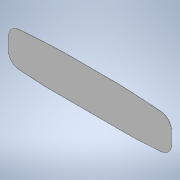
# Autodesk Inventor part: 7 Segment Clock Shell
Saved by Autodesk Inventor 2021 (Build 250183000, 183)
## iProperties
Created: 2020-06-27
Part Number: 7 Segment Clock Shell
Material: Generic
Document SubType Name: Modeling
Designer: dech3
Density: 1 g/cm^3
Appearance: Default
Author: dech3
Autodesk Inventor part; units mm, degrees
ref_plane "YZ Plane" through (0, 0, 0) normal (1, 0, 0) x (0, 1, 0)
ref_plane "XZ Plane" through (0, 0, 0) normal (0, 1, 0) x (-1, 0, 0)
ref_plane "XY Plane" through (0, 0, 0) normal (0, 0, 1) x (1, 0, 0)
sketch "Block1" plane through (0, 0, 0) normal (0, 0, 1) x (1, 0, 0)
  arc A0 (261.5609, 58.5131) -> (100.3256, 67.9894) centre (0, -3015.4231) ccw
  arc A1 (-100.3256, 67.9894) -> (-261.5609, 58.5131) centre (0, -3015.4231) ccw
  line L0 (-159.5034, -75) -> (159.5034, -75)
  arc A2 (-263.2612, -68.2167) -> (-160.4975, -74.9753) centre (0, 3150) ccw
  arc A3 (160.4975, -74.9753) -> (263.2612, -68.2167) centre (0, 3150) ccw
  arc A4 (300, 16.6643) -> (261.5609, 58.5131) centre (258, 16.6643) ccw
  arc A5 (263.2612, -68.2167) -> (300, -28.3498) centre (260, -28.3498) ccw
  arc A6 (-300, -28.3498) -> (-263.2612, -68.2167) centre (-260, -28.3498) ccw
  arc A7 (-261.5609, 58.5131) -> (-300, 16.6643) centre (-258, 16.6643) ccw
  arc A8 (-99.6752, 68) -> (-100.3256, 67.9894) centre (-99.6752, 48) ccw
  arc A9 (100.3256, 67.9894) -> (99.6752, 68) centre (99.6752, 48) ccw
  arc A10 (159.5034, -75) -> (160.4975, -74.9753) centre (159.5034, -55) ccw
  arc A11 (-160.4975, -74.9753) -> (-159.5034, -75) centre (-159.5034, -55) ccw
  line L1 (-99.6752, 68) -> (99.6752, 68)
  line L2 (300, 16.6643) -> (300, -28.3498)
  line L3 (-300, -28.3498) -> (-300, 16.6643)
  point P0 (0, -2.2582)
  point P1 (-300, 55)
  point P2 (300, 55)
  point P3 (-300, -65)
  point P4 (300, -65)
  point P5 (-160, -75)
  point P6 (160, -75)
  point P7 (-100, 68)
  point P8 (100, 68)
  dimension "d0" = 600
  dimension "d14" = 120
  dimension "d13" = 120
  dimension "d12" = 140
  dimension "d10" = 140
  dimension "d3" = 200
  dimension "d1" = 200
  dimension "d20" = 200
  dimension "d21" = 320
  dimension "d2" = 143
  dimension "d11" = 10
  dimension "d9" = 10
  dimension "d22" = 13
  dimension "d23" = 13
  dimension "d8" = 42
  dimension "d7" = 40
  dimension "d6" = 40
  dimension "d5" = 42
  dimension "d4" = 20
  measures "d0" distance between parallel lines of L2 L3
  measures "d14" distance of point (-300, 55) point (-300, -65)
  measures "d13" distance of point (300, 55) point (300, -65)
  measures "d12" horizontal distance of point (-300, -65) point (-160, -75)
  measures "d10" horizontal distance of point (300, -65) point (160, -75)
  measures "d3" horizontal distance of point (-300, 55) point (-100, 68)
  measures "d1" horizontal distance of point (300, 55) point (100, 68)
  measures "d20" distance of point (100, 68) point (-100, 68)
  measures "d21" distance of point (160, -75) point (-160, -75)
  measures "d2" distance from line of L0 point (-100, 68)
  measures "d11" vertical distance of point (-300, -65) point (-160, -75)
  measures "d9" vertical distance of point (300, -65) point (160, -75)
  measures "d22" vertical distance of point (100, 68) point (300, 55)
  measures "d23" vertical distance of point (-100, 68) point (-300, 55)
  measures "d8" radius of A4
  measures "d7" radius of A5
  measures "d6" radius of A6
  measures "d5" radius of A7
  measures "d4" radius of A8
sketch "Sketch2" plane through (0, 0, 0) normal (0, 0, 1) x (1, 0, 0)
  arc A0 (261.5609, 58.5131) -> (100.3256, 67.9894) centre (0, -3015.4231) ccw
  arc A1 (-100.3256, 67.9894) -> (-261.5609, 58.5131) centre (0, -3015.4231) ccw
  line L0 (-159.5034, -75) -> (159.5034, -75)
  arc A2 (-263.2612, -68.2167) -> (-160.4975, -74.9753) centre (0, 3150) ccw
  arc A3 (160.4975, -74.9753) -> (263.2612, -68.2167) centre (0, 3150) ccw
  arc A4 (300, 16.6643) -> (261.5609, 58.5131) centre (258, 16.6643) ccw
  arc A5 (263.2612, -68.2167) -> (300, -28.3498) centre (260, -28.3498) ccw
  arc A6 (-300, -28.3498) -> (-263.2612, -68.2167) centre (-260, -28.3498) ccw
  arc A7 (-261.5609, 58.5131) -> (-300, 16.6643) centre (-258, 16.6643) ccw
  arc A8 (-99.6752, 68) -> (-100.3256, 67.9894) centre (-99.6752, 48) ccw
  arc A9 (100.3256, 67.9894) -> (99.6752, 68) centre (99.6752, 48) ccw
  arc A10 (159.5034, -75) -> (160.4975, -74.9753) centre (159.5034, -55) ccw
  arc A11 (-160.4975, -74.9753) -> (-159.5034, -75) centre (-159.5034, -55) ccw
  line L1 (-99.6752, 68) -> (99.6752, 68)
  line L2 (300, 16.6643) -> (300, -28.3498)
  line L3 (-300, -28.3498) -> (-300, 16.6643)
  point P0 (0, 0)
  point P1 (0, 0)
  dimension "d16" = 300
  dimension "d15" = 75
extrude "Extrusion1" add sketch "Sketch2" along normal blind 0.5
body "Solid1"
